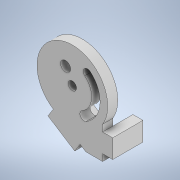
# Autodesk Inventor part: mutato_segéd
Saved by Autodesk Inventor 2020 (Build 240168000, 168)
## iProperties
Created: 2019-09-19
Part Number: mutato_segéd
Material: Generic
Document SubType Name: Modeling
Designer: Horváth Patrik
Density: 1 g/cm^3
Appearance: Default
Author: Horváth Patrik
Autodesk Inventor part; units mm, degrees
ref_plane "YZ Plane" through (0, 0, 0) normal (1, 0, 0) x (0, 1, 0)
ref_plane "XZ Plane" through (0, 0, 0) normal (0, 1, 0) x (-1, 0, 0)
ref_plane "XY Plane" through (0, 0, 0) normal (0, 0, 1) x (1, 0, 0)
sketch "Sketch1" plane through (0, 0, 0) normal (0, 0, 1) x (1, 0, 0)
  line L0 (9, -5.4083) -> (2.8559, -8.0613) construction
  circle A0 centre (0, 0) radius 1.25
  circle A1 centre (-2, 4) radius 1.5
  circle A2 centre (0, 0) radius 1.25 construction
  arc A3 (3.5, -6.0622) -> (4.4995, 5.3623) centre (0, 0) ccw construction
  arc A4 (4.125, -7.1447) -> (5.303, 6.3199) centre (0, 0) ccw
  arc A5 (2.875, -4.9796) -> (3.696, 4.4048) centre (0, 0) ccw
  arc A6 (2.875, -4.9796) -> (4.125, -7.1447) centre (3.5, -6.0622) ccw
  arc A7 (5.303, 6.3199) -> (3.696, 4.4048) centre (4.4995, 5.3623) ccw
  line L1 (4.4995, 5.3623) -> (0, 0) construction
  line L2 (0, 0) -> (7, 0) construction
  line L3 (0, 0) -> (3.5, -6.0622) construction
  line L4 (9, -5.4083) -> (2.8559, -8.0613) construction
  arc A8 (9, -5.4083) -> (-5.6429, -8.8548) centre (0, 0) ccw
  line L5 (4, -15) -> (9, -15)
  line L6 (9, -5.4083) -> (9, -15)
  line L7 (9, 0) -> (4, 0)
  line L8 (4, -15) -> (-5.6429, -8.8548)
  line L9 (-17.5314, 0) -> (16.8044, 0) construction
  line L10 (0, -20.5253) -> (0, 18.1516) construction
  dimension "d0" = 3
  dimension "d1" = 4
  dimension "d2" = 2
  dimension "d3" = 2.5
  dimension "d4" = 50
  dimension "d5" = 60
  dimension "d6" = 7
  dimension "d7" = 2.5
  dimension "d8" = 15
  dimension "d10" = 10.5
  dimension "d11" = 5
  dimension "d12" = 9
  constraints: 18 end point, 14 point on circle, 9 centre point, 5 tangent, 4 coincident, 2 parallel, 1 collinear, 1 concentric, 1 horizontal, 1 point on line
  measures "d0" diameter of A1
  measures "d1" vertical distance of A0.centre A1.centre
  measures "d2" horizontal distance of A0.centre A1.centre
  measures "d3" radial gap between concentric circles of A4 A5
  measures "d4" angle of L2 L1
  measures "d5" angle of L3 L2
  measures "d6" radius of A3
  measures "d7" diameter of A0
  measures "d8" distance from line of L2.end L5
  measures "d10" radius of A8
  measures "d11" distance of L5.start L5.end
  measures "d12" distance from line of L6 point (0, 0)
extrude "Extrusion1" add sketch "Sketch1" along normal blind 3
sketch "Sketch2" plane through (0, 0, 3) normal (0, 0, 1) x (1, 0, 0)
  line L0 (-5.6429, -8.8548) -> (4, -15) construction
  line L1 (9, -15) -> (9, -5.4083) construction
  line L2 (-5.6429, -8.8548) -> (4, -15) construction
  line L3 (4, -15) -> (9, -15) construction
  line L4 (9, -15) -> (9, -5.4083) construction
  arc A0 (9, -5.4083) -> (-5.6429, -8.8548) centre (0, 0) ccw construction
  arc A1 (5.303, 6.3199) -> (3.696, 4.4048) centre (4.4995, 5.3623) ccw construction
  arc A2 (4.125, -7.1447) -> (5.303, 6.3199) centre (0, 0) ccw construction
  arc A3 (2.875, -4.9796) -> (4.125, -7.1447) centre (3.5, -6.0622) ccw construction
  arc A4 (2.875, -4.9796) -> (3.696, 4.4048) centre (0, 0) ccw construction
  circle A5 centre (0, 0) radius 1.25 construction
  circle A6 centre (-2, 4) radius 1.5 construction
  line L5 (-5.6429, -8.8548) -> (2.3134, -13.9252)
  line L6 (2.3134, -13.9252) -> (0.7011, -16.4551)
  line L7 (0.7011, -16.4551) -> (-7.2552, -11.3847)
  line L8 (-7.2552, -11.3847) -> (-5.6429, -8.8548)
  line L9 (9, -13) -> (9, -7.4083)
  line L10 (9, -7.4083) -> (12, -7.4083)
  line L11 (12, -7.4083) -> (12, -13)
  line L12 (12, -13) -> (9, -13)
  dimension "d15" = 3
  dimension "d16" = 3
  dimension "d17" = 2
  dimension "d18" = 2
  dimension "d19" = 2
  constraints: 16 end point, 4 parallel, 3 point on line, 2 perpendicular
  measures "d15" distance between parallel lines of L0 L7
  measures "d16" distance between parallel lines of L1 L11
  measures "d17" distance from line of L6 L0.end
  measures "d18" distance between parallel lines of L3 L12
  measures "d19" distance from line of L1.end L10
extrude "Extrusion2" add sketch "Sketch2" against normal blind 9
sketch "Sketch3" plane through (0, 0, 0) normal (0, 0, -1) x (-1, 0, 0)
  line L0 (5.6429, -8.8548) -> (-2.3134, -13.9252) construction
  arc A0 (5.6429, -8.8548) -> (-9, -5.4083) centre (0, 0) ccw construction
  line L1 (-9, -7.4083) -> (-9, -5.4083) construction
  line L2 (-9, -13) -> (-9, -7.4083) construction
  line L3 (-9, -15) -> (-9, -13) construction
  line L4 (-4, -15) -> (-9, -15) construction
  line L5 (-2.3134, -13.9252) -> (-4, -15) construction
  arc A1 (-3.696, 4.4048) -> (-5.303, 6.3199) centre (-4.4995, 5.3623) ccw construction
  arc A2 (-3.696, 4.4048) -> (-2.875, -4.9796) centre (0, 0) ccw construction
  arc A3 (-4.125, -7.1447) -> (-2.875, -4.9796) centre (-3.5, -6.0622) ccw construction
  arc A4 (-5.303, 6.3199) -> (-4.125, -7.1447) centre (0, 0) ccw construction
  circle A5 centre (0, 0) radius 1.25 construction
  circle A6 centre (2, 4) radius 1.5 construction
  circle A7 centre (0, 0) radius 1.25 projected
  arc A8 (3, -5.1962) -> (6, 0) centre (0, 0) ccw construction
  arc A9 (5.6429, -8.8548) -> (10.5, 0) centre (0, 0) ccw
  arc A10 (0.8061, -1.265) -> (1.5, 0) centre (0, 0) ccw
  line L6 (0.8061, -1.265) -> (5.6429, -8.8548)
  line L7 (10.5, 0) -> (1.5, 0)
  dimension "d22" = 9
  constraints: 6 point on circle, 4 end point, 3 centre point, 2 horizontal alignment, 1 coincident, 1 concentric, 1 horizontal, 1 point on line
  measures "d22" radial gap between concentric circles of A0 A10
extrude "Extrusion3" add sketch "Sketch3" along normal blind 3 contours L6 A10 L7 A9
equation "\"d16\" = d15"
body "Solid1"
